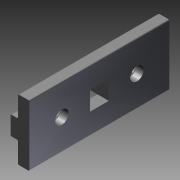
# Autodesk Inventor part: 6705_p
Saved by Autodesk Inventor 2011 SP1 (Build 150282100, 282)
## iProperties
Created: 2017-08-19
Part Number: 6705_p
Catalog Web Link: www.cadenas.de
Description: 6705, 6706, 6814, 6817_p-UniBearing Bearing Pads
Vendor: 8020
Document SubType Name: Modeling
Designer: psAdmin
Manufacturer: 8020
Mass: 3.82398 g
Surface Area: 27.465 cm^2
Volume: 3.82398 cm^3
Density: 1 g/cm^3
Category: PARTsolutions
Company: 8020
Title: 6705_p
Author: Cadenas PARTsolutions
Comments: UniBearing Bearing Pads
PSOL_IDENT_0: {$CADENAS_DATA\23d-libs\8020\inch\linear_motion\6705.prj},172 {VTYP=3D},{NB=6705_p},{LINA=6705_p},{N
PSOL_IDENT_1: N=6705, 6706, 6814, 6817_p},{DATE=21.08.2013 15:58:18},{GEOMDATE=16.03.2012 00:00:00},{VERSION=},{LI
PSOL_IDENT_2: NEID=10},{LINESUBID=-1},{WBVAR=}  {NB=6705_p},{LINA=6705_p},{KT=DUMMY},{PN=6705},{COLOR=White},{COL=
PSOL_IDENT_3: 1.00,1.00,1.00,0.00},{A=0.812},{B=0.406},{C=0.432},{D=1.865},{E=1.000},{F=0.100},{G=0.250},{H=.250 ±
PSOL_IDENT_4: .003},{H1=0.250},{J=.150 ± .003},{J1=0.150},{K=#8-32},{K1=0.164},{W=.010},{CB=0.332},{CBD=0.088},{H
PSOL_IDENT_5: D1=0.177},{SH=0.250},{NO=1},{SCR=8-32}
NN: 6705, 6706, 6814, 6817_p
NT: UniBearing Bearing Pads
NB: 6705_p
NBSYN: $PN._p
LINA: 6705_p
PN: 6705
COLOR: White
A: 0.812
B: 0.406
C: 0.432
D: 1.865
E: 1.000
F: 0.100
G: 0.250
H: .250 ± .003
H1: 0.250
J: .150 ± .003
J1: 0.150
K: #8-32
K1: 0.164
W: .010
CB: 0.332
CBD: 0.088
HD1: 0.177
SH: 0.250
NO: 1
SCR: 8-32
SUPPLIER: 8020
ARTICLENO: 6705_p
BOMINFO: 6705_p
CREATOR: CADENAS GmbH
Autodesk Inventor part; units mm, degrees
ref_plane "YZ Plane" through (0, 0, 0) normal (1, 0, 0) x (0, 1, 0)
ref_plane "XZ Plane" through (0, 0, 0) normal (0, 1, 0) x (-1, 0, 0)
ref_plane "XY Plane" through (0, 0, 0) normal (0, 0, 1) x (1, 0, 0)
sketch "Sketch_1" plane through (0, 0, 0) normal (0, 0, 1) x (1, 0, 0)
  line L0 (-6.35, 2.794) -> (-6.35, -2.794)
  arc A0 (-6.35, -2.794) -> (-5.969, -3.175) centre (-5.969, -2.794) ccw
  line L1 (-5.969, -3.175) -> (-4.191, -3.175)
  arc A1 (-3.81, -3.556) -> (-4.191, -3.175) centre (-4.191, -3.556) ccw
  line L2 (-3.81, -3.556) -> (-3.81, -9.9314)
  arc A2 (-3.81, -9.9314) -> (-3.429, -10.3124) centre (-3.429, -9.9314) ccw
  line L3 (-3.429, -10.3124) -> (-0.381, -10.3124)
  arc A3 (-0.381, -10.3124) -> (0, -9.9314) centre (-0.381, -9.9314) ccw
  line L4 (0, -9.9314) -> (0, 9.9314)
  arc A4 (0, 9.9314) -> (-0.381, 10.3124) centre (-0.381, 9.9314) ccw
  line L5 (-0.381, 10.3124) -> (-3.429, 10.3124)
  arc A5 (-3.429, 10.3124) -> (-3.81, 9.9314) centre (-3.429, 9.9314) ccw
  line L6 (-3.81, 9.9314) -> (-3.81, 3.556)
  arc A6 (-4.191, 3.175) -> (-3.81, 3.556) centre (-4.191, 3.556) ccw
  line L7 (-4.191, 3.175) -> (-5.969, 3.175)
  arc A7 (-5.969, 3.175) -> (-6.35, 2.794) centre (-5.969, 2.794) ccw
  constraints: 16 end point, 16 point on circle, 8 centre point
extrude "Extrusion1" add sketch "Sketch_1" along normal mid plane 47.371
sketch "Sketch_2" plane through (0, 0, 12.7) normal (0, 0, 1) x (1, 0, 0)
  line L0 (0, 0) -> (-6.35, 0)
  line L1 (-6.35, 0) -> (-6.35, 4.2164)
  line L2 (-6.35, 4.2164) -> (-4.1148, 4.2164)
  line L3 (-4.1148, 4.2164) -> (-2.463, 2.2479)
  line L4 (-2.463, 2.2479) -> (0, 2.2479)
  line L5 (0, 2.2479) -> (0, 0)
  line L6 (0, 0) -> (-6.35, 0)
  constraints: 14 end point
revolve "Revolution1" cut sketch "Sketch_2" angle 360 about axis through (0, 0, 12.7) along (1, 0, 0)
sketch "Sketch_3" plane through (0, 0, -12.7) normal (0, 0, 1) x (1, 0, 0)
  line L0 (0, 0) -> (-6.35, 0)
  line L1 (-6.35, 0) -> (-6.35, 4.2164)
  line L2 (-6.35, 4.2164) -> (-4.1148, 4.2164)
  line L3 (-4.1148, 4.2164) -> (-2.463, 2.2479)
  line L4 (-2.463, 2.2479) -> (0, 2.2479)
  line L5 (0, 2.2479) -> (0, 0)
  line L6 (0, 0) -> (-6.35, 0)
  constraints: 14 end point
revolve "Revolution2" cut sketch "Sketch_3" angle 360 about axis through (0, 0, -12.7) along (1, 0, 0)
sketch "Sketch_4" plane through (0, 0, 0) normal (1, 0, 0) x (0, 1, 0)
  line L0 (-3.175, 3.175) -> (-3.175, -3.175)
  line L1 (-3.175, -3.175) -> (3.175, -3.175)
  line L2 (3.175, -3.175) -> (3.175, 3.175)
  line L3 (3.175, 3.175) -> (-3.175, 3.175)
  constraints: 8 end point
extrude "Extrusion2" cut sketch "Sketch_4" against normal blind 6.35
sketch "Sketch_5" plane through (0, 0, 0) normal (0, 0, 1) x (1, 0, 0)
  line L0 (-10.16, 6.35) -> (-10.16, -6.35)
  line L1 (-10.16, -6.35) -> (-3.81, -6.35)
  line L2 (-3.81, -6.35) -> (-3.81, 6.35)
  line L3 (-3.81, 6.35) -> (-10.16, 6.35)
  constraints: 8 end point
extrude "Extrusion3" cut sketch "Sketch_5" along normal mid plane 6.35
ref_plane "pad_XY" through (0, 0, -12.7) normal (1, 0, 0) x (0, 0, -1)
ref_plane "pad_YZ" through (0, 0, -12.7) normal (0, 0, -1) x (0, 1, 0)
ref_plane "pad_ZX" through (0, 0, -12.7) normal (0, 1, 0) x (1, 0, 0)
ref_plane "s1_XY" through (-2.463, 0, 12.7) normal (1, 0, 0) x (0, 0, -1)
ref_plane "s1_YZ" through (-2.463, 0, 12.7) normal (0, 0, -1) x (0, 1, 0)
ref_plane "s1_ZX" through (-2.463, 0, 12.7) normal (0, 1, 0) x (1, 0, 0)
ref_plane "s2_XY" through (-2.463, 0, -12.7) normal (1, 0, 0) x (0, 0, -1)
ref_plane "s2_YZ" through (-2.463, 0, -12.7) normal (0, 0, -1) x (0, 1, 0)
ref_plane "s2_ZX" through (-2.463, 0, -12.7) normal (0, 1, 0) x (1, 0, 0)
body "Solid1"
